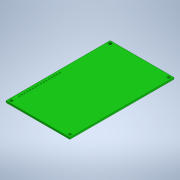
# Autodesk Inventor part: Mounting_PCB
Saved by Autodesk Inventor 2020 (Build 240168000, 168)
## iProperties
Created: 2020-11-23
Part Number: Mounting_PCB
Material: Generic
Document SubType Name: Modeling
Designer: nico
Density: 1 g/cm^3
Appearance: Dark Green
Author: nico
Autodesk Inventor part; units mm, degrees
ref_plane "YZ Plane" through (0, 0, 0) normal (1, 0, 0) x (0, 1, 0)
ref_plane "XZ Plane" through (0, 0, 0) normal (0, 1, 0) x (-1, 0, 0)
ref_plane "XY Plane" through (0, 0, 0) normal (0, 0, 1) x (1, 0, 0)
sketch "PCB" plane through (0, 0, 0) normal (0, 1, 0) x (-1, 0, 0)
  line L0 (0, 0) -> (60, 0)
  line L1 (60, 0) -> (60, -98)
  line L2 (60, -98) -> (0, -98)
  line L3 (0, -98) -> (0, 0)
  dimension "d0" = 98
  dimension "d1" = 60
  constraints: 8 end point, 2 parallel, 1 horizontal, 1 perpendicular
  measures "d0" distance between parallel lines of L2 L0
  measures "d1" distance between parallel lines of L3 L1
extrude "PCB_Extr" add sketch "PCB" along normal blind 1.6
sketch "Mounting" plane through (0, 1.6, 0) normal (0, 1, 0) x (1, 0, 0)
  circle A0 centre (-57.5, 2.5) radius 1.25
  circle A1 centre (-57.5, 95.5) radius 1.25
  circle A2 centre (-2.5, 95.5) radius 1.25
  circle A3 centre (-2.5, 2.5) radius 1.25
  line L0 (-60, 0) -> (0, 0) projected
  line L1 (-60, 98) -> (-60, 0) projected
  line L2 (0, 98) -> (-60, 98) projected
  line L3 (0, 0) -> (0, 98) projected
  dimension "d4" = 2.5
  dimension "d5" = 2.5
  dimension "d6" = 2.5
  dimension "d7" = 2.5
  dimension "d8" = 2.5
  dimension "d9" = 2.5
  dimension "d10" = 2.5
  dimension "d11" = 2.5
  dimension "d12" = 2.5
  dimension "d13" = 2.5
  dimension "d14" = 2.5
  dimension "d15" = 2.5
  constraints: 4 centre point
  measures "d4" diameter of A0
  measures "d5" diameter of A1
  measures "d6" diameter of A2
  measures "d7" diameter of A3
  measures "d8" distance from line of L0 A0.centre
  measures "d9" distance from line of L1 A0.centre
  measures "d10" distance from line of L1 A1.centre
  measures "d11" distance from line of L2 A1.centre
  measures "d12" distance from line of L2 A2.centre
  measures "d13" distance from line of L3 A2.centre
  measures "d14" distance from line of L0 A3.centre
  measures "d15" distance from line of L3 A3.centre
extrude "Mounting_Extr" cut sketch "Mounting" against normal through all contours A0 | A1 | A2 | A3
sketch "Pinning" plane through (0, 1.6, 0) normal (0, 1, 0) x (1, 0, 0)
  circle A0 centre (-57.5, 10) radius 0.5
  circle A1 centre (-57.5, 12.54) radius 0.5
  circle A2 centre (-57.5, 15.08) radius 0.5
  circle A3 centre (-57.5, 25.24) radius 0.5
  circle A4 centre (-57.5, 20.16) radius 0.5
  circle A5 centre (-57.5, 27.78) radius 0.5
  circle A6 centre (-57.5, 22.7) radius 0.5
  circle A7 centre (-57.5, 17.62) radius 0.5
  line L0 (-60, 0) -> (0, 0) projected
  line L1 (-60, 98) -> (-60, 0) projected
  line L2 (-59.0965, 29.05) -> (-55.5485, 29.05)
  circle A8 centre (-57.5, 48.1) radius 0.5
  circle A9 centre (-57.5, 45.56) radius 0.5
  circle A10 centre (-57.5, 43.02) radius 0.5
  circle A11 centre (-57.5, 32.86) radius 0.5
  circle A12 centre (-57.5, 37.94) radius 0.5
  circle A13 centre (-57.5, 30.32) radius 0.5
  circle A14 centre (-57.5, 35.4) radius 0.5
  circle A15 centre (-57.5, 40.48) radius 0.5
  dimension "d18" = 1
  dimension "d19" = 1
  dimension "d20" = 1
  dimension "d21" = 1
  dimension "d22" = 1
  dimension "d23" = 1
  dimension "d24" = 1
  dimension "d25" = 1
  dimension "d26" = 10
  dimension "d27" = 2.5
  dimension "d28" = 2.54
  dimension "d29" = 2.54
  dimension "d30" = 2.54
  dimension "d31" = 2.54
  dimension "d32" = 2.54
  dimension "d33" = 2.54
  dimension "d34" = 2.54
  dimension "d38" = 1.27
  constraints: 16 centre point, 8 symmetric about line, 7 vertical alignment, 2 end point, 1 horizontal, 8 other
  measures "d18" diameter of A0
  measures "d19" diameter of A1
  measures "d20" diameter of A2
  measures "d21" diameter of A3
  measures "d22" diameter of A4
  measures "d23" diameter of A5
  measures "d24" diameter of A6
  measures "d25" diameter of A7
  measures "d26" distance from line of L0 A0.centre
  measures "d27" distance from line of L1 A0.centre
  measures "d28" distance of A1.centre A0.centre
  measures "d29" distance of A2.centre A1.centre
  measures "d30" distance of A7.centre A2.centre
  measures "d31" distance of A4.centre A7.centre
  measures "d32" distance of A4.centre A6.centre
  measures "d33" distance of A6.centre A3.centre
  measures "d34" distance of A3.centre A5.centre
  measures "d38" distance from line of A5.centre L2
extrude "Pinning_Extr" cut sketch "Pinning" against normal through all
equation "\"d5\" = d4"
equation "\"d6\" = d4"
equation "\"d7\" = d4"
equation "\"d9\" = d8"
equation "\"d10\" = d8"
equation "\"d11\" = d8"
equation "\"d12\" = d8"
equation "\"d13\" = d8"
equation "\"d14\" = d8"
equation "\"d15\" = d8"
equation "\"d19\" = d18"
equation "\"d20\" = d18"
equation "\"d21\" = d18"
equation "\"d22\" = d18"
equation "\"d23\" = d18"
equation "\"d24\" = d18"
equation "\"d25\" = d18"
equation "\"d29\" = d28"
equation "\"d30\" = d28"
equation "\"d31\" = d28"
equation "\"d32\" = d28"
equation "\"d33\" = d28"
equation "\"d34\" = d28"
body "Solid1"
